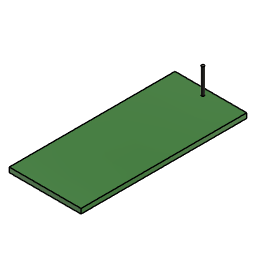
Assembly CanSat - ASCENT Lite v1.0.0 v11 (Autodesk Fusion 360 archive; units mm, degrees)
design "Telemetrie (in scheiße) v1.0.0"
Autodesk Fusion 360 part; units mm, degrees
sketch "Skizze1" plane through (0, 0, 0) normal (0, 0, 1) x (1, 0, 0)
  line L0 (-40, -20) -> (-16.1, -20)
  line L1 (-16.1, -20) -> (-16.1, 35.2)
  line L2 (-16.1, 35.2) -> (-40, 35.2)
  line L3 (-40, 35.2) -> (-40, -20)
  dimension "d1" = 23.9
  dimension "d2" = 55.2
  constraint horizontal L0
  constraint vertical L1
  constraint horizontal L2
  constraint vertical L3
  measures "d1" distance of L0.start L0.end
  measures "d2" distance of L0 L2
extrude "Extrusion1" add sketch "Skizze1" along normal blind 1.6 makes body 1
sketch "Skizze2" plane through (0, 0, 1.6) normal (0, 0, 1) x (-1, 0, 0)
  line L0 (40, -35.2) -> (40, 20)
  line L1 (40, 20) -> (16.1, 20)
  line L2 (16.1, 20) -> (16.1, -35.2)
  line L3 (16.1, -35.2) -> (40, -35.2)
  circle A0 centre (28.5, -33) radius 0.5
  dimension "d5" = 1
  measures "d5" diameter of A0
extrude "Extrusion2" add sketch "Skizze2" along normal blind 8.5 separate body contours A0 makes body 2
copy_body "Körper->Berechn3" bodies 2 removing the originals makes body 3 in component "Component'"
copy_body "Körper->Berechn4" bodies 1 removing the originals makes body 4 in component "Component''"
component "Component'" placed x (1, 0, 0) y (0, 1, 0) z (0, 0, 1) at (0, 0, 0)
component "Component''" placed x (1, 0, 0) y (0, 1, 0) z (0, 0, 1) at (0, 0, 0)

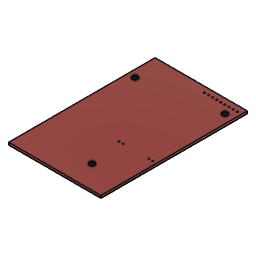
design "EAGLE (in scheiße) v1.0.0"
Autodesk Fusion 360 part; units mm, degrees
sketch "Skizze1" plane through (0, 0, 0) normal (0, 0, 1) x (1, 0, 0)
  line L0 (-60.2435, -23.188) -> (-3.1435, -23.188)
  line L1 (-3.1435, -23.188) -> (-3.1435, 67.512)
  line L2 (-3.1435, 67.512) -> (-60.2435, 67.512)
  line L3 (-60.2435, 67.512) -> (-60.2435, -23.188)
  dimension "d1" = 57.1
  dimension "d2" = 90.7
  constraint horizontal L0
  constraint vertical L1
  constraint horizontal L2
  constraint vertical L3
  measures "d1" distance of L0.start L0.end
  measures "d2" distance of L0 L2
extrude "Extrusion1" add sketch "Skizze1" along normal blind 1.5
sketch "Skizze2" plane through (0, 0, 1.5) normal (0, 0, 1) x (-1, 0, 0)
  line L0 (60.2435, -67.512) -> (60.2435, 23.188)
  line L1 (60.2435, 23.188) -> (3.1435, 23.188)
  line L2 (3.1435, 23.188) -> (3.1435, -67.512)
  line L3 (3.1435, -67.512) -> (60.2435, -67.512)
  line L4 (4.5435, -65.382) -> (27.5435, -65.382)
  line L5 (27.5435, -65.382) -> (27.5435, -62.722)
  line L6 (27.5435, -62.722) -> (4.5435, -62.722)
  line L7 (4.5435, -62.722) -> (4.5435, -65.382)
  line L8 (9.3435, -10.062) -> (4.1435, -10.062)
  line L9 (4.1435, -10.062) -> (4.1435, -12.722)
  line L10 (4.1435, -12.722) -> (9.3435, -12.722)
  line L11 (9.3435, -12.722) -> (9.3435, -10.062)
  circle A0 centre (5.8735, -64) radius 0.5
  circle A1 centre (8.4135, -64) radius 0.5
  circle A2 centre (10.9535, -64) radius 0.5
  circle A3 centre (13.4935, -64) radius 0.5
  circle A4 centre (16.0335, -64) radius 0.5
  circle A5 centre (18.5735, -64) radius 0.5
  circle A6 centre (21.1135, -64) radius 0.5
  circle A7 centre (23.6535, -64) radius 0.5
  circle A8 centre (26.1935, -64) radius 0.5
  circle A9 centre (5.4735, -11.3967) radius 0.5
  circle A10 centre (8.0135, -11.3967) radius 0.5
  circle A11 centre (23.9735, -11.3967) radius 0.5
  line L12 (27.8435, -12.722) -> (27.8435, -10.062)
  circle A12 centre (26.5135, -11.3967) radius 0.5
  line L13 (22.6435, -10.062) -> (22.6435, -12.722)
  line L14 (27.8435, -10.062) -> (22.6435, -10.062)
  line L15 (22.6435, -12.722) -> (27.8435, -12.722)
  dimension "d5" = 23
  dimension "d6" = 2.66
  dimension "d7" = 1.4
  dimension "d8" = 2.13
  dimension "d11" = 5.2
  dimension "d12" = 2.66
  dimension "d13" = 50
  dimension "d14" = 1
  dimension "d17" = 1
  dimension "d20" = 2.54
  dimension "d21" = 0
  dimension "d22" = 1.33
  dimension "d23" = 1
  dimension "d26" = 2.54
  dimension "d27" = 0
  dimension "d28" = 1.33
  dimension "d31" = 2.54
  dimension "d32" = 0
  dimension "d33" = 5.2
  dimension "d34" = 2.66
  dimension "d35" = 1
  dimension "d36" = 1.33
  dimension "d37" = 13.3
  constraint horizontal L4
  constraint vertical L5
  constraint horizontal L6
  constraint vertical L7
  constraint horizontal L10
  constraint vertical L11
  constraint horizontal L8
  constraint vertical L9
  constraint horizontal L15
  constraint vertical L12
  constraint horizontal L14
  constraint vertical L13
  measures "d5" distance of L4.start L4.end
  measures "d6" distance of L4 L6
  measures "d7" distance of L2 L7
  measures "d8" distance of L3 L4
  measures "d11" distance of L9.end L10.end
  measures "d12" distance of L8 L10
  measures "d13" distance of L6 L10
  measures "d14" distance of L2 L9
  measures "d17" diameter of A0
  measures "d22" distance of L7 A0.centre
  measures "d23" diameter of A9
  measures "d28" distance of L9 A9.centre
  measures "d33" distance of L13.end L12.start
  measures "d34" distance of L14 L15
  measures "d35" diameter of A11
  measures "d36" distance of A11.centre L13
  measures "d37" distance of L11 L13
extrude "Extrusion2" cut sketch "Skizze2" along normal through all and the other way through all contours A0 | A1 | A2 | A3 | A4 | A5 | A6 | A7 | A8 | A9 | A10 | A11 | A12
sketch "Skizze3" plane through (0, 0, 1.5) normal (0, 0, 1) x (-1, 0, 0)
  circle A0 centre (23.9735, -11.3967) radius 0.5
  circle A1 centre (21.1135, -64) radius 0.5
  circle A2 centre (10.9535, -64) radius 0.5
  circle A3 centre (8.4135, -64) radius 0.5
  circle A4 centre (18.5735, -64) radius 0.5
  circle A5 centre (26.5135, -11.3967) radius 0.5
  circle A6 centre (8.0135, -11.3967) radius 0.5
  circle A7 centre (23.6535, -64) radius 0.5
  circle A8 centre (13.4935, -64) radius 0.5
  circle A9 centre (5.8735, -64) radius 0.5
  circle A10 centre (16.0335, -64) radius 0.5
  circle A11 centre (26.1935, -64) radius 0.5
  circle A12 centre (5.4735, -11.3967) radius 0.5
  line L0 (60.2435, -67.512) -> (60.2435, 23.188)
  line L1 (60.2435, 23.188) -> (3.1435, 23.188)
  line L2 (3.1435, 23.188) -> (3.1435, -67.512)
  line L3 (3.1435, -67.512) -> (60.2435, -67.512)
  circle A13 centre (8.3735, -58.912) radius 1.6
  circle A14 centre (55.6435, -50.512) radius 1.6
  circle A15 centre (22.7935, 8.988) radius 1.6
  dimension "d40" = 3.2
  dimension "d41" = 3.2
  dimension "d42" = 3.2
  dimension "d43" = 8.6
  dimension "d44" = 5.23
  dimension "d45" = 17
  dimension "d46" = 4.6
  dimension "d47" = 14.2
  dimension "d48" = 19.65
  measures "d40" diameter of A13
  measures "d41" diameter of A14
  measures "d42" diameter of A15
  measures "d43" distance of L3 A13.centre
  measures "d44" distance of L2 A13.centre
  measures "d45" distance of L3 A14.centre
  measures "d46" distance of L0 A14.centre
  measures "d47" distance of L1 A15.centre
  measures "d48" distance of L2 A15.centre
extrude "Extrusion3" cut sketch "Skizze3" along normal mid plane 8 contours A13 | A14 | A15

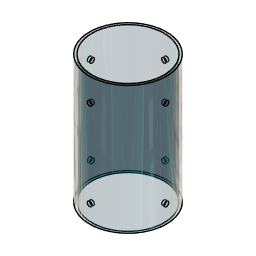
design "Mantel v1"
Autodesk Fusion 360 part; units mm, degrees
sketch "Skizze1" plane through (0, 0, 0) normal (0, 0, 1) x (1, 0, 0)
  circle A0 centre (0, 0) radius 33
  circle A1 centre (0, 0) radius 31
  dimension "d1" = 66
  dimension "d2" = 62
  constraint coincident A0.centre A1.centre
  measures "d1" diameter of A0
  measures "d2" diameter of A1
extrude "Extrusion1" add sketch "Skizze1" along normal blind 110
ref_plane "Arbeitsebene1" through (0, -33, 66.517) normal (0, -1, 0) x (-1, 0, 0)
sketch "Skizze2" plane through (0, -33, 0) normal (0, -1, 0) x (-1, 0, 0)
  circle A0 centre (0, -15) radius 2
  line L0 (-33, 0) -> (33, 0)
  circle A1 centre (0, -89.878) radius 2
  dimension "d6" = 4
  dimension "d7" = 15
  dimension "d8" = 4
  dimension "d9" = 89.878
  measures "d6" diameter of A0
  measures "d7" distance of A0.centre L0
  measures "d8" diameter of A1
  measures "d9" distance of L0 A1.centre
extrude "Extrusion2" cut sketch "Skizze2" against normal blind 70
pattern_circular "C-Anordnung1" count 4 over 360 about axis through (0, 0, 0) along (0, 0, 1) of "Extrusion2"
equation "d9 = 89.3 mm + 0.578 mm"

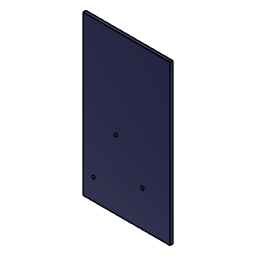
design "Sensorik (in Scheiße) v1.0.0"
Autodesk Fusion 360 part; units mm, degrees
sketch "Skizze1" plane through (0, 0, 0) normal (0, 1, 0) x (1, 0, 0)
  line L0 (-60, 20) -> (-5.3, 20)
  line L1 (-5.3, 20) -> (-5.3, -79.8)
  line L2 (-5.3, -79.8) -> (-60, -79.8)
  line L3 (-60, -79.8) -> (-60, 20)
  dimension "d1" = 54.7
  dimension "d2" = 99.8
  constraint horizontal L0
  constraint vertical L1
  constraint horizontal L2
  constraint vertical L3
  measures "d1" distance of L0.start L0.end
  measures "d2" distance of L0 L2
extrude "Extrusion1" add sketch "Skizze1" along normal blind 1.8
sketch "Skizze2" plane through (0, 1.8, 0) normal (0, 1, 0) x (-1, 0, 0)
  line L0 (60, 79.8) -> (5.3, 79.8)
  line L1 (5.3, 79.8) -> (5.3, -20)
  line L2 (5.3, -20) -> (60, -20)
  line L3 (60, -20) -> (60, 79.8)
  circle A0 centre (22.7, 2.6) radius 1
  circle A1 centre (53.43, -6.85) radius 1
  circle A2 centre (39.36, 23.2) radius 1
  dimension "d5" = 2
  dimension "d6" = 2
  dimension "d7" = 2
  dimension "d8" = 22.6
  dimension "d9" = 17.4
  dimension "d10" = 13.15
  dimension "d11" = 6.57
  dimension "d12" = 20.64
  dimension "d13" = 43.2
  measures "d5" diameter of A0
  measures "d6" diameter of A1
  measures "d7" diameter of A2
  measures "d8" distance of L2 A0.centre
  measures "d9" distance of L1 A0.centre
  measures "d10" distance of L2 A1.centre
  measures "d11" distance of L3 A1.centre
  measures "d12" distance of L3 A2.centre
  measures "d13" distance of L2 A2.centre
extrude "Extrusion3" cut sketch "Skizze2" against normal blind 4 contours A0 | A1 | A2
extrude "Extrusion2" [suppressed]
